Autodesk Inventor part; units mm, degrees
(part 4 of 13)
  arc A1197 (1.0789, 60.921) -> (1.0789, 60.795) centre (1.0789, 60.858) ccw
  line L1196 (7.637, 60.795) -> (7.7628, 60.795)
  arc A1198 (7.7628, 60.795) -> (7.7628, 60.921) centre (7.7628, 60.858) ccw
  line L1197 (7.7628, 60.921) -> (7.637, 60.921)
  arc A1199 (7.637, 60.921) -> (7.637, 60.795) centre (7.637, 60.858) ccw
  line L1198 (8.7151, 60.795) -> (17.121, 60.795)
  arc A1200 (17.121, 60.795) -> (17.121, 60.921) centre (17.121, 60.858) ccw
  line L1199 (17.121, 60.921) -> (8.7151, 60.921)
  arc A1201 (8.7151, 60.921) -> (8.7151, 60.795) centre (8.7151, 60.858) ccw
  line L1200 (1.0789, 60.921) -> (6.8108, 60.921)
  arc A1202 (6.8108, 60.921) -> (6.8108, 61.047) centre (6.8108, 60.984) ccw
  line L1201 (6.8108, 61.047) -> (1.0789, 61.047)
  arc A1203 (1.0789, 61.047) -> (1.0789, 60.921) centre (1.0789, 60.984) ccw
  line L1202 (7.637, 60.921) -> (7.7628, 60.921)
  arc A1204 (7.7628, 60.921) -> (7.7628, 61.047) centre (7.7628, 60.984) ccw
  line L1203 (7.7628, 61.047) -> (7.637, 61.047)
  arc A1205 (7.637, 61.047) -> (7.637, 60.921) centre (7.637, 60.984) ccw
  line L1204 (8.5891, 60.921) -> (17.121, 60.921)
  arc A1206 (17.121, 60.921) -> (17.121, 61.047) centre (17.121, 60.984) ccw
  line L1205 (17.121, 61.047) -> (8.5891, 61.047)
  arc A1207 (8.5891, 61.047) -> (8.5891, 60.921) centre (8.5891, 60.984) ccw
  line L1206 (1.0789, 61.047) -> (6.9527, 61.047)
  arc A1208 (6.9527, 61.047) -> (6.9527, 61.173) centre (6.9527, 61.11) ccw
  line L1207 (6.9527, 61.173) -> (1.0789, 61.173)
  arc A1209 (1.0789, 61.173) -> (1.0789, 61.047) centre (1.0789, 61.11) ccw
  line L1208 (7.637, 61.047) -> (7.7628, 61.047)
  arc A1210 (7.7628, 61.047) -> (7.7628, 61.173) centre (7.7628, 61.11) ccw
  line L1209 (7.7628, 61.173) -> (7.637, 61.173)
  arc A1211 (7.637, 61.173) -> (7.637, 61.047) centre (7.637, 61.11) ccw
  line L1210 (8.4473, 61.047) -> (17.121, 61.047)
  arc A1212 (17.121, 61.047) -> (17.121, 61.173) centre (17.121, 61.11) ccw
  line L1211 (17.121, 61.173) -> (8.4473, 61.173)
  arc A1213 (8.4473, 61.173) -> (8.4473, 61.047) centre (8.4473, 61.11) ccw
  line L1212 (1.0789, 61.173) -> (7.2569, 61.173)
  arc A1214 (7.2569, 61.173) -> (7.2569, 61.299) centre (7.2569, 61.236) ccw
  line L1213 (7.2569, 61.299) -> (1.0789, 61.299)
  arc A1215 (1.0789, 61.299) -> (1.0789, 61.173) centre (1.0789, 61.236) ccw
  line L1214 (7.637, 61.173) -> (7.7628, 61.173)
  arc A1216 (7.7628, 61.173) -> (7.7628, 61.299) centre (7.7628, 61.236) ccw
  line L1215 (7.7628, 61.299) -> (7.637, 61.299)
  arc A1217 (7.637, 61.299) -> (7.637, 61.173) centre (7.637, 61.236) ccw
  line L1216 (8.1431, 61.173) -> (17.121, 61.173)
  arc A1218 (17.121, 61.173) -> (17.121, 61.299) centre (17.121, 61.236) ccw
  line L1217 (17.121, 61.299) -> (8.1431, 61.299)
  arc A1219 (8.1431, 61.299) -> (8.1431, 61.173) centre (8.1431, 61.236) ccw
  line L1218 (1.0789, 61.299) -> (17.121, 61.299)
  arc A1220 (17.121, 61.299) -> (17.121, 61.425) centre (17.121, 61.362) ccw
  line L1219 (17.121, 61.425) -> (1.0789, 61.425)
  arc A1221 (1.0789, 61.425) -> (1.0789, 61.299) centre (1.0789, 61.362) ccw
  line L1220 (1.0789, 61.425) -> (17.121, 61.425)
  arc A1222 (17.121, 61.425) -> (17.121, 61.551) centre (17.121, 61.488) ccw
  line L1221 (17.121, 61.551) -> (1.0789, 61.551)
  arc A1223 (1.0789, 61.551) -> (1.0789, 61.425) centre (1.0789, 61.488) ccw
  line L1222 (1.0789, 61.551) -> (17.121, 61.551)
  arc A1224 (17.121, 61.551) -> (17.121, 61.677) centre (17.121, 61.614) ccw
  line L1223 (17.121, 61.677) -> (1.0789, 61.677)
  arc A1225 (1.0789, 61.677) -> (1.0789, 61.551) centre (1.0789, 61.614) ccw
  line L1224 (1.0789, 61.677) -> (17.121, 61.677)
  arc A1226 (17.121, 61.677) -> (17.121, 61.803) centre (17.121, 61.74) ccw
  line L1225 (17.121, 61.803) -> (1.0789, 61.803)
  arc A1227 (1.0789, 61.803) -> (1.0789, 61.677) centre (1.0789, 61.74) ccw
  line L1226 (1.0789, 61.803) -> (17.121, 61.803)
  arc A1228 (17.121, 61.803) -> (17.121, 61.929) centre (17.121, 61.866) ccw
  line L1227 (17.121, 61.929) -> (1.0789, 61.929)
  arc A1229 (1.0789, 61.929) -> (1.0789, 61.803) centre (1.0789, 61.866) ccw
  line L1228 (1.0789, 61.929) -> (17.121, 61.929)
  arc A1230 (17.121, 61.929) -> (17.121, 62.055) centre (17.121, 61.992) ccw
  line L1229 (17.121, 62.055) -> (1.0789, 62.055)
  arc A1231 (1.0789, 62.055) -> (1.0789, 61.929) centre (1.0789, 61.992) ccw
  line L1230 (1.0789, 62.055) -> (17.121, 62.055)
  arc A1232 (17.121, 62.055) -> (17.121, 62.181) centre (17.121, 62.118) ccw
  line L1231 (17.121, 62.181) -> (1.0789, 62.181)
  arc A1233 (1.0789, 62.181) -> (1.0789, 62.055) centre (1.0789, 62.118) ccw
  line L1232 (1.0789, 62.181) -> (17.121, 62.181)
  arc A1234 (17.121, 62.181) -> (17.121, 62.307) centre (17.121, 62.244) ccw
  line L1233 (17.121, 62.307) -> (1.0789, 62.307)
  arc A1235 (1.0789, 62.307) -> (1.0789, 62.181) centre (1.0789, 62.244) ccw
  line L1234 (1.0789, 62.307) -> (17.121, 62.307)
  arc A1236 (17.121, 62.307) -> (17.121, 62.433) centre (17.121, 62.37) ccw
  line L1235 (17.121, 62.433) -> (1.0789, 62.433)
  arc A1237 (1.0789, 62.433) -> (1.0789, 62.307) centre (1.0789, 62.37) ccw
  line L1236 (1.0789, 62.433) -> (17.121, 62.433)
  arc A1238 (17.121, 62.433) -> (17.121, 62.559) centre (17.121, 62.496) ccw
  line L1237 (17.121, 62.559) -> (1.0789, 62.559)
  arc A1239 (1.0789, 62.559) -> (1.0789, 62.433) centre (1.0789, 62.496) ccw
  line L1238 (1.0789, 62.559) -> (17.121, 62.559)
  arc A1240 (17.121, 62.559) -> (17.121, 62.685) centre (17.121, 62.622) ccw
  line L1239 (17.121, 62.685) -> (1.0789, 62.685)
  arc A1241 (1.0789, 62.685) -> (1.0789, 62.559) centre (1.0789, 62.622) ccw
  line L1240 (1.0789, 62.685) -> (17.121, 62.685)
  arc A1242 (17.121, 62.685) -> (17.121, 62.811) centre (17.121, 62.748) ccw
  line L1241 (17.121, 62.811) -> (1.0789, 62.811)
  arc A1243 (1.0789, 62.811) -> (1.0789, 62.685) centre (1.0789, 62.748) ccw
  line L1242 (1.0789, 62.811) -> (17.121, 62.811)
  arc A1244 (17.121, 62.811) -> (17.121, 62.937) centre (17.121, 62.874) ccw
  line L1243 (17.121, 62.937) -> (1.0789, 62.937)
  arc A1245 (1.0789, 62.937) -> (1.0789, 62.811) centre (1.0789, 62.874) ccw
  line L1244 (1.0789, 62.937) -> (17.121, 62.937)
  arc A1246 (17.121, 62.937) -> (17.121, 63.063) centre (17.121, 63) ccw
  line L1245 (17.121, 63.063) -> (1.0789, 63.063)
  arc A1247 (1.0789, 63.063) -> (1.0789, 62.937) centre (1.0789, 63) ccw
  line L1246 (1.0789, 63.063) -> (17.121, 63.063)
  arc A1248 (17.121, 63.063) -> (17.121, 63.189) centre (17.121, 63.126) ccw
  line L1247 (17.121, 63.189) -> (1.0789, 63.189)
  arc A1249 (1.0789, 63.189) -> (1.0789, 63.063) centre (1.0789, 63.126) ccw
  line L1248 (17.058, 63.221) -> (17.058, 1.0789)
  arc A1250 (17.058, 1.0789) -> (17.184, 1.0789) centre (17.121, 1.0789) ccw
  line L1249 (17.184, 1.0789) -> (17.184, 63.221)
  arc A1251 (17.184, 63.221) -> (17.058, 63.221) centre (17.121, 63.221) ccw
  line L1250 (17.121, 1.1419) -> (1.0789, 1.1419)
  arc A1252 (1.0789, 1.1419) -> (1.0789, 1.0159) centre (1.0789, 1.0789) ccw
  line L1251 (1.0789, 1.0159) -> (17.121, 1.0159)
  arc A1253 (17.121, 1.0159) -> (17.121, 1.1419) centre (17.121, 1.0789) ccw
  line L1252 (1.1419, 1.0789) -> (1.1419, 63.221)
  arc A1254 (1.1419, 63.221) -> (1.0159, 63.221) centre (1.0789, 63.221) ccw
  line L1253 (1.0159, 63.221) -> (1.0159, 1.0789)
  arc A1255 (1.0159, 1.0789) -> (1.1419, 1.0789) centre (1.0789, 1.0789) ccw
  line L1254 (1.0789, 63.158) -> (17.121, 63.158)
  arc A1256 (17.121, 63.158) -> (17.121, 63.284) centre (17.121, 63.221) ccw
  line L1255 (17.121, 63.284) -> (1.0789, 63.284)
  arc A1257 (1.0789, 63.284) -> (1.0789, 63.158) centre (1.0789, 63.221) ccw
  line L1256 (7.428, 58.51) -> (7.637, 58.51)
  arc A1258 (7.637, 58.51) -> (7.637, 58.636) centre (7.637, 58.573) ccw
  line L1257 (7.637, 58.636) -> (7.428, 58.636)
  arc A1259 (7.428, 58.636) -> (7.428, 58.51) centre (7.428, 58.573) ccw
  line L1258 (7.7, 58.573) -> (7.7, 59.8765)
  arc A1260 (7.7, 59.8765) -> (7.574, 59.8765) centre (7.637, 59.8765) ccw
  line L1259 (7.574, 59.8765) -> (7.574, 58.573)
  arc A1261 (7.574, 58.573) -> (7.7, 58.573) centre (7.637, 58.573) ccw
  line L1260 (7.637, 59.8135) -> (7.7628, 59.8135)
  arc A1262 (7.7628, 59.8135) -> (7.7628, 59.9395) centre (7.7628, 59.8765) ccw
  line L1261 (7.7628, 59.9395) -> (7.637, 59.9395)
  arc A1263 (7.637, 59.9395) -> (7.637, 59.8135) centre (7.637, 59.8765) ccw
  line L1262 (7.6998, 59.8765) -> (7.6998, 58.573)
  arc A1264 (7.6998, 58.573) -> (7.8258, 58.573) centre (7.7628, 58.573) ccw
  line L1263 (7.8258, 58.573) -> (7.8258, 59.8765)
  arc A1265 (7.8258, 59.8765) -> (7.6998, 59.8765) centre (7.7628, 59.8765) ccw
  line L1264 (7.7628, 58.51) -> (7.9719, 58.51)
  arc A1266 (7.9719, 58.51) -> (7.9719, 58.636) centre (7.9719, 58.573) ccw
  line L1265 (7.9719, 58.636) -> (7.7628, 58.636)
  arc A1267 (7.7628, 58.636) -> (7.7628, 58.51) centre (7.7628, 58.573) ccw
  line L1266 (7.996, 58.5148) -> (8.4984, 58.7229)
  arc A1268 (8.4984, 58.7229) -> (8.4502, 58.8393) centre (8.4743, 58.7811) ccw
  line L1267 (8.4502, 58.8393) -> (7.9478, 58.6312)
  arc A1269 (7.9478, 58.6312) -> (7.996, 58.5148) centre (7.9719, 58.573) ccw
  line L1268 (8.5188, 58.7366) -> (8.9033, 59.1211)
  arc A1270 (8.9033, 59.1211) -> (8.8143, 59.2101) centre (8.8588, 59.1656) ccw
  line L1269 (8.8143, 59.2101) -> (8.4298, 58.8256)
  arc A1271 (8.4298, 58.8256) -> (8.5188, 58.7366) centre (8.4743, 58.7811) ccw
  line L1270 (8.917, 59.1415) -> (9.1251, 59.6439)
  arc A1272 (9.1251, 59.6439) -> (9.0087, 59.6921) centre (9.0669, 59.668) ccw
  line L1271 (9.0087, 59.6921) -> (8.8006, 59.1897)
  arc A1273 (8.8006, 59.1897) -> (8.917, 59.1415) centre (8.8588, 59.1656) ccw
  line L1272 (9.1299, 59.668) -> (9.1299, 59.877)
  arc A1274 (9.1299, 59.877) -> (9.0039, 59.877) centre (9.0669, 59.877) ccw
  line L1273 (9.0039, 59.877) -> (9.0039, 59.668)
  arc A1275 (9.0039, 59.668) -> (9.1299, 59.668) centre (9.0669, 59.668) ccw
  line L1274 (9.0669, 59.94) -> (7.7634, 59.94)
  arc A1276 (7.7634, 59.94) -> (7.7634, 59.814) centre (7.7634, 59.877) ccw
  line L1275 (7.7634, 59.814) -> (9.0669, 59.814)
  arc A1277 (9.0669, 59.814) -> (9.0669, 59.94) centre (9.0669, 59.877) ccw
  line L1276 (7.8264, 59.877) -> (7.8264, 60.0028)
  arc A1278 (7.8264, 60.0028) -> (7.7004, 60.0028) centre (7.7634, 60.0028) ccw
  line L1277 (7.7004, 60.0028) -> (7.7004, 59.877)
  arc A1279 (7.7004, 59.877) -> (7.8264, 59.877) centre (7.7634, 59.877) ccw
  line L1278 (7.7634, 59.9398) -> (9.0669, 59.9398)
  arc A1280 (9.0669, 59.9398) -> (9.0669, 60.0658) centre (9.0669, 60.0028) ccw
  line L1279 (9.0669, 60.0658) -> (7.7634, 60.0658)
  arc A1281 (7.7634, 60.0658) -> (7.7634, 59.9398) centre (7.7634, 60.0028) ccw
  line L1280 (9.1299, 60.0028) -> (9.1299, 60.2119)
  arc A1282 (9.1299, 60.2119) -> (9.0039, 60.2119) centre (9.0669, 60.2119) ccw
  line L1281 (9.0039, 60.2119) -> (9.0039, 60.0028)
  arc A1283 (9.0039, 60.0028) -> (9.1299, 60.0028) centre (9.0669, 60.0028) ccw
  line L1282 (9.1251, 60.236) -> (8.917, 60.7384)
  arc A1284 (8.917, 60.7384) -> (8.8006, 60.6902) centre (8.8588, 60.7143) ccw
  line L1283 (8.8006, 60.6902) -> (9.0087, 60.1878)
  arc A1285 (9.0087, 60.1878) -> (9.1251, 60.236) centre (9.0669, 60.2119) ccw
  line L1284 (8.9033, 60.7588) -> (8.5188, 61.1433)
  arc A1286 (8.5188, 61.1433) -> (8.4298, 61.0543) centre (8.4743, 61.0988) ccw
  line L1285 (8.4298, 61.0543) -> (8.8143, 60.6698)
  arc A1287 (8.8143, 60.6698) -> (8.9033, 60.7588) centre (8.8588, 60.7143) ccw
  line L1286 (8.4984, 61.157) -> (7.996, 61.3651)
  arc A1288 (7.996, 61.3651) -> (7.9478, 61.2487) centre (7.9719, 61.3069) ccw
  line L1287 (7.9478, 61.2487) -> (8.4502, 61.0406)
  arc A1289 (8.4502, 61.0406) -> (8.4984, 61.157) centre (8.4743, 61.0988) ccw
  line L1288 (7.9719, 61.3699) -> (7.7628, 61.3699)
  arc A1290 (7.7628, 61.3699) -> (7.7628, 61.2439) centre (7.7628, 61.3069) ccw
  line L1289 (7.7628, 61.2439) -> (7.9719, 61.2439)
  arc A1291 (7.9719, 61.2439) -> (7.9719, 61.3699) centre (7.9719, 61.3069) ccw
  line L1290 (7.6998, 61.3069) -> (7.6998, 60.0034)
  arc A1292 (7.6998, 60.0034) -> (7.8258, 60.0034) centre (7.7628, 60.0034) ccw
  line L1291 (7.8258, 60.0034) -> (7.8258, 61.3069)
  arc A1293 (7.8258, 61.3069) -> (7.6998, 61.3069) centre (7.7628, 61.3069) ccw
  line L1292 (7.7628, 60.0664) -> (7.637, 60.0664)
  arc A1294 (7.637, 60.0664) -> (7.637, 59.9404) centre (7.637, 60.0034) ccw
  line L1293 (7.637, 59.9404) -> (7.7628, 59.9404)
  arc A1295 (7.7628, 59.9404) -> (7.7628, 60.0664) centre (7.7628, 60.0034) ccw
  line L1294 (7.7, 60.0034) -> (7.7, 61.3069)
  arc A1296 (7.7, 61.3069) -> (7.574, 61.3069) centre (7.637, 61.3069) ccw
  line L1295 (7.574, 61.3069) -> (7.574, 60.0034)
  arc A1297 (7.574, 60.0034) -> (7.7, 60.0034) centre (7.637, 60.0034) ccw
  line L1296 (7.637, 61.3699) -> (7.428, 61.3699)
  arc A1298 (7.428, 61.3699) -> (7.428, 61.2439) centre (7.428, 61.3069) ccw
  line L1297 (7.428, 61.2439) -> (7.637, 61.2439)
  arc A1299 (7.637, 61.2439) -> (7.637, 61.3699) centre (7.637, 61.3069) ccw
  line L1298 (7.4039, 61.3651) -> (6.9015, 61.157)
  arc A1300 (6.9015, 61.157) -> (6.9497, 61.0406) centre (6.9256, 61.0988) ccw
  line L1299 (6.9497, 61.0406) -> (7.4521, 61.2487)
  arc A1301 (7.4521, 61.2487) -> (7.4039, 61.3651) centre (7.428, 61.3069) ccw
  line L1300 (6.8811, 61.1433) -> (6.4966, 60.7588)
  arc A1302 (6.4966, 60.7588) -> (6.5856, 60.6698) centre (6.5411, 60.7143) ccw
  line L1301 (6.5856, 60.6698) -> (6.9701, 61.0543)
  arc A1303 (6.9701, 61.0543) -> (6.8811, 61.1433) centre (6.9256, 61.0988) ccw
  line L1302 (6.4829, 60.7384) -> (6.2748, 60.236)
  arc A1304 (6.2748, 60.236) -> (6.3912, 60.1878) centre (6.333, 60.2119) ccw
  line L1303 (6.3912, 60.1878) -> (6.5993, 60.6902)
  arc A1305 (6.5993, 60.6902) -> (6.4829, 60.7384) centre (6.5411, 60.7143) ccw
  line L1304 (6.27, 60.2119) -> (6.27, 60.0028)
  arc A1306 (6.27, 60.0028) -> (6.396, 60.0028) centre (6.333, 60.0028) ccw
  line L1305 (6.396, 60.0028) -> (6.396, 60.2119)
  arc A1307 (6.396, 60.2119) -> (6.27, 60.2119) centre (6.333, 60.2119) ccw
  line L1306 (6.333, 59.9398) -> (7.6365, 59.9398)
  arc A1308 (7.6365, 59.9398) -> (7.6365, 60.0658) centre (7.6365, 60.0028) ccw
  line L1307 (7.6365, 60.0658) -> (6.333, 60.0658)
  arc A1309 (6.333, 60.0658) -> (6.333, 59.9398) centre (6.333, 60.0028) ccw
  line L1308 (7.5735, 60.0028) -> (7.5735, 59.877)
  arc A1310 (7.5735, 59.877) -> (7.6995, 59.877) centre (7.6365, 59.877) ccw
  line L1309 (7.6995, 59.877) -> (7.6995, 60.0028)
  arc A1311 (7.6995, 60.0028) -> (7.5735, 60.0028) centre (7.6365, 60.0028) ccw
  line L1310 (7.6365, 59.94) -> (6.333, 59.94)
  arc A1312 (6.333, 59.94) -> (6.333, 59.814) centre (6.333, 59.877) ccw
  line L1311 (6.333, 59.814) -> (7.6365, 59.814)
  arc A1313 (7.6365, 59.814) -> (7.6365, 59.94) centre (7.6365, 59.877) ccw
  line L1312 (6.27, 59.877) -> (6.27, 59.668)
  arc A1314 (6.27, 59.668) -> (6.396, 59.668) centre (6.333, 59.668) ccw
  line L1313 (6.396, 59.668) -> (6.396, 59.877)
  arc A1315 (6.396, 59.877) -> (6.27, 59.877) centre (6.333, 59.877) ccw
  line L1314 (6.2748, 59.6439) -> (6.4829, 59.1415)
  arc A1316 (6.4829, 59.1415) -> (6.5993, 59.1897) centre (6.5411, 59.1656) ccw
  line L1315 (6.5993, 59.1897) -> (6.3912, 59.6921)
  arc A1317 (6.3912, 59.6921) -> (6.2748, 59.6439) centre (6.333, 59.668) ccw
  line L1316 (6.4966, 59.1211) -> (6.8811, 58.7366)
  arc A1318 (6.8811, 58.7366) -> (6.9701, 58.8256) centre (6.9256, 58.7811) ccw
  line L1317 (6.9701, 58.8256) -> (6.5856, 59.2101)
  arc A1319 (6.5856, 59.2101) -> (6.4966, 59.1211) centre (6.5411, 59.1656) ccw
  line L1318 (6.9015, 58.7229) -> (7.4039, 58.5148)
  arc A1320 (7.4039, 58.5148) -> (7.4521, 58.6312) centre (7.428, 58.573) ccw
  line L1319 (7.4521, 58.6312) -> (6.9497, 58.8393)
  arc A1321 (6.9497, 58.8393) -> (6.9015, 58.7229) centre (6.9256, 58.7811) ccw
  line L1320 (9.0283, 54.6082) -> (9.0283, 55.1117)
  arc A1322 (9.0283, 55.1117) -> (8.9023, 55.1117) centre (8.9653, 55.1117) ccw
  line L1321 (8.9023, 55.1117) -> (8.9023, 54.6082)
  arc A1323 (8.9023, 54.6082) -> (9.0283, 54.6082) centre (8.9653, 54.6082) ccw
  line L1322 (9.0235, 55.1358) -> (8.8309, 55.6008)
  arc A1324 (8.8309, 55.6008) -> (8.7145, 55.5526) centre (8.7727, 55.5767) ccw
  line L1323 (8.7145, 55.5526) -> (8.9071, 55.0876)
  arc A1325 (8.9071, 55.0876) -> (9.0235, 55.1358) centre (8.9653, 55.1117) ccw
  line L1324 (8.8172, 55.6212) -> (8.4612, 55.9772)
  arc A1326 (8.4612, 55.9772) -> (8.3722, 55.8882) centre (8.4167, 55.9327) ccw
  line L1325 (8.3722, 55.8882) -> (8.7282, 55.5322)
  arc A1327 (8.7282, 55.5322) -> (8.8172, 55.6212) centre (8.7727, 55.5767) ccw
  line L1326 (8.4408, 55.9909) -> (7.9758, 56.1835)
  arc A1328 (7.9758, 56.1835) -> (7.9276, 56.0671) centre (7.9517, 56.1253) ccw
  line L1327 (7.9276, 56.0671) -> (8.3926, 55.8745)
  arc A1329 (8.3926, 55.8745) -> (8.4408, 55.9909) centre (8.4167, 55.9327) ccw
  line L1328 (7.9517, 56.1883) -> (7.4482, 56.1883)
  arc A1330 (7.4482, 56.1883) -> (7.4482, 56.0623) centre (7.4482, 56.1253) ccw
  line L1329 (7.4482, 56.0623) -> (7.9517, 56.0623)
  arc A1331 (7.9517, 56.0623) -> (7.9517, 56.1883) centre (7.9517, 56.1253) ccw
  line L1330 (7.4241, 56.1835) -> (6.9591, 55.9909)
  arc A1332 (6.9591, 55.9909) -> (7.0073, 55.8745) centre (6.9832, 55.9327) ccw
  line L1331 (7.0073, 55.8745) -> (7.4723, 56.0671)
  arc A1333 (7.4723, 56.0671) -> (7.4241, 56.1835) centre (7.4482, 56.1253) ccw
  line L1332 (6.9387, 55.9772) -> (6.5827, 55.6212)
  arc A1334 (6.5827, 55.6212) -> (6.6717, 55.5322) centre (6.6272, 55.5767) ccw
  line L1333 (6.6717, 55.5322) -> (7.0277, 55.8882)
  arc A1335 (7.0277, 55.8882) -> (6.9387, 55.9772) centre (6.9832, 55.9327) ccw
  line L1334 (6.569, 55.6008) -> (6.3764, 55.1358)
  arc A1336 (6.3764, 55.1358) -> (6.4928, 55.0876) centre (6.4346, 55.1117) ccw
  line L1335 (6.4928, 55.0876) -> (6.6854, 55.5526)
  arc A1337 (6.6854, 55.5526) -> (6.569, 55.6008) centre (6.6272, 55.5767) ccw
  line L1336 (6.3716, 55.1117) -> (6.3716, 54.6082)
  arc A1338 (6.3716, 54.6082) -> (6.4976, 54.6082) centre (6.4346, 54.6082) ccw
  line L1337 (6.4976, 54.6082) -> (6.4976, 55.1117)
  arc A1339 (6.4976, 55.1117) -> (6.3716, 55.1117) centre (6.4346, 55.1117) ccw
  line L1338 (6.3764, 54.5841) -> (6.569, 54.1191)
  arc A1340 (6.569, 54.1191) -> (6.6854, 54.1673) centre (6.6272, 54.1432) ccw
  line L1339 (6.6854, 54.1673) -> (6.4928, 54.6323)
  arc A1341 (6.4928, 54.6323) -> (6.3764, 54.5841) centre (6.4346, 54.6082) ccw
  line L1340 (6.5827, 54.0987) -> (6.9387, 53.7427)
  arc A1342 (6.9387, 53.7427) -> (7.0277, 53.8317) centre (6.9832, 53.7872) ccw
  line L1341 (7.0277, 53.8317) -> (6.6717, 54.1877)
  arc A1343 (6.6717, 54.1877) -> (6.5827, 54.0987) centre (6.6272, 54.1432) ccw
  line L1342 (6.9591, 53.729) -> (7.4241, 53.5364)
  arc A1344 (7.4241, 53.5364) -> (7.4723, 53.6528) centre (7.4482, 53.5946) ccw
  line L1343 (7.4723, 53.6528) -> (7.0073, 53.8454)
  arc A1345 (7.0073, 53.8454) -> (6.9591, 53.729) centre (6.9832, 53.7872) ccw
  line L1344 (7.4482, 53.5316) -> (7.9517, 53.5316)
  arc A1346 (7.9517, 53.5316) -> (7.9517, 53.6576) centre (7.9517, 53.5946) ccw
  line L1345 (7.9517, 53.6576) -> (7.4482, 53.6576)
  arc A1347 (7.4482, 53.6576) -> (7.4482, 53.5316) centre (7.4482, 53.5946) ccw
  line L1346 (7.9758, 53.5364) -> (8.4408, 53.729)
  arc A1348 (8.4408, 53.729) -> (8.3926, 53.8454) centre (8.4167, 53.7872) ccw
  line L1347 (8.3926, 53.8454) -> (7.9276, 53.6528)
  arc A1349 (7.9276, 53.6528) -> (7.9758, 53.5364) centre (7.9517, 53.5946) ccw
  line L1348 (8.4612, 53.7427) -> (8.8172, 54.0987)
  arc A1350 (8.8172, 54.0987) -> (8.7282, 54.1877) centre (8.7727, 54.1432) ccw
  line L1349 (8.7282, 54.1877) -> (8.3722, 53.8317)
  arc A1351 (8.3722, 53.8317) -> (8.4612, 53.7427) centre (8.4167, 53.7872) ccw
  line L1350 (8.8309, 54.1191) -> (9.0235, 54.5841)
  arc A1352 (9.0235, 54.5841) -> (8.9071, 54.6323) centre (8.9653, 54.6082) ccw
  line L1351 (8.9071, 54.6323) -> (8.7145, 54.1673)
  arc A1353 (8.7145, 54.1673) -> (8.8309, 54.1191) centre (8.7727, 54.1432) ccw
  line L1352 (7.428, 38.19) -> (7.637, 38.19)
  arc A1354 (7.637, 38.19) -> (7.637, 38.316) centre (7.637, 38.253) ccw
  line L1353 (7.637, 38.316) -> (7.428, 38.316)
  arc A1355 (7.428, 38.316) -> (7.428, 38.19) centre (7.428, 38.253) ccw
  line L1354 (7.7, 38.253) -> (7.7, 39.5565)
  arc A1356 (7.7, 39.5565) -> (7.574, 39.5565) centre (7.637, 39.5565) ccw
  line L1355 (7.574, 39.5565) -> (7.574, 38.253)
  arc A1357 (7.574, 38.253) -> (7.7, 38.253) centre (7.637, 38.253) ccw
  line L1356 (7.637, 39.4935) -> (7.7628, 39.4935)
  arc A1358 (7.7628, 39.4935) -> (7.7628, 39.6195) centre (7.7628, 39.5565) ccw
  line L1357 (7.7628, 39.6195) -> (7.637, 39.6195)
  arc A1359 (7.637, 39.6195) -> (7.637, 39.4935) centre (7.637, 39.5565) ccw
  line L1358 (7.6998, 39.5565) -> (7.6998, 38.253)
  arc A1360 (7.6998, 38.253) -> (7.8258, 38.253) centre (7.7628, 38.253) ccw
  line L1359 (7.8258, 38.253) -> (7.8258, 39.5565)
  arc A1361 (7.8258, 39.5565) -> (7.6998, 39.5565) centre (7.7628, 39.5565) ccw
  line L1360 (7.7628, 38.19) -> (7.9719, 38.19)
  arc A1362 (7.9719, 38.19) -> (7.9719, 38.316) centre (7.9719, 38.253) ccw
  line L1361 (7.9719, 38.316) -> (7.7628, 38.316)
  arc A1363 (7.7628, 38.316) -> (7.7628, 38.19) centre (7.7628, 38.253) ccw
  line L1362 (7.996, 38.1948) -> (8.4984, 38.4029)
  arc A1364 (8.4984, 38.4029) -> (8.4502, 38.5193) centre (8.4743, 38.4611) ccw
  line L1363 (8.4502, 38.5193) -> (7.9478, 38.3112)
  arc A1365 (7.9478, 38.3112) -> (7.996, 38.1948) centre (7.9719, 38.253) ccw
  line L1364 (8.5188, 38.4166) -> (8.9033, 38.8011)
  arc A1366 (8.9033, 38.8011) -> (8.8143, 38.8901) centre (8.8588, 38.8456) ccw
  line L1365 (8.8143, 38.8901) -> (8.4298, 38.5056)
  arc A1367 (8.4298, 38.5056) -> (8.5188, 38.4166) centre (8.4743, 38.4611) ccw
  line L1366 (8.917, 38.8215) -> (9.1251, 39.3239)
  arc A1368 (9.1251, 39.3239) -> (9.0087, 39.3721) centre (9.0669, 39.348) ccw
  line L1367 (9.0087, 39.3721) -> (8.8006, 38.8697)
  arc A1369 (8.8006, 38.8697) -> (8.917, 38.8215) centre (8.8588, 38.8456) ccw
  line L1368 (9.1299, 39.348) -> (9.1299, 39.557)
  arc A1370 (9.1299, 39.557) -> (9.0039, 39.557) centre (9.0669, 39.557) ccw
  line L1369 (9.0039, 39.557) -> (9.0039, 39.348)
  arc A1371 (9.0039, 39.348) -> (9.1299, 39.348) centre (9.0669, 39.348) ccw
  line L1370 (9.0669, 39.62) -> (7.7634, 39.62)
  arc A1372 (7.7634, 39.62) -> (7.7634, 39.494) centre (7.7634, 39.557) ccw
  line L1371 (7.7634, 39.494) -> (9.0669, 39.494)
  arc A1373 (9.0669, 39.494) -> (9.0669, 39.62) centre (9.0669, 39.557) ccw
  line L1372 (7.8264, 39.557) -> (7.8264, 39.6828)
  arc A1374 (7.8264, 39.6828) -> (7.7004, 39.6828) centre (7.7634, 39.6828) ccw
  line L1373 (7.7004, 39.6828) -> (7.7004, 39.557)
  arc A1375 (7.7004, 39.557) -> (7.8264, 39.557) centre (7.7634, 39.557) ccw
  line L1374 (7.7634, 39.6198) -> (9.0669, 39.6198)
  arc A1376 (9.0669, 39.6198) -> (9.0669, 39.7458) centre (9.0669, 39.6828) ccw
  line L1375 (9.0669, 39.7458) -> (7.7634, 39.7458)
  arc A1377 (7.7634, 39.7458) -> (7.7634, 39.6198) centre (7.7634, 39.6828) ccw
  line L1376 (9.1299, 39.6828) -> (9.1299, 39.8919)
  arc A1378 (9.1299, 39.8919) -> (9.0039, 39.8919) centre (9.0669, 39.8919) ccw
  line L1377 (9.0039, 39.8919) -> (9.0039, 39.6828)
  arc A1379 (9.0039, 39.6828) -> (9.1299, 39.6828) centre (9.0669, 39.6828) ccw
  line L1378 (9.1251, 39.916) -> (8.917, 40.4184)
  arc A1380 (8.917, 40.4184) -> (8.8006, 40.3702) centre (8.8588, 40.3943) ccw
  line L1379 (8.8006, 40.3702) -> (9.0087, 39.8678)
  arc A1381 (9.0087, 39.8678) -> (9.1251, 39.916) centre (9.0669, 39.8919) ccw
  line L1380 (8.9033, 40.4388) -> (8.5188, 40.8233)
  arc A1382 (8.5188, 40.8233) -> (8.4298, 40.7343) centre (8.4743, 40.7788) ccw
  line L1381 (8.4298, 40.7343) -> (8.8143, 40.3498)
  arc A1383 (8.8143, 40.3498) -> (8.9033, 40.4388) centre (8.8588, 40.3943) ccw
  line L1382 (8.4984, 40.837) -> (7.996, 41.0451)
  arc A1384 (7.996, 41.0451) -> (7.9478, 40.9287) centre (7.9719, 40.9869) ccw
  line L1383 (7.9478, 40.9287) -> (8.4502, 40.7206)
  arc A1385 (8.4502, 40.7206) -> (8.4984, 40.837) centre (8.4743, 40.7788) ccw
  line L1384 (7.9719, 41.0499) -> (7.7628, 41.0499)
  arc A1386 (7.7628, 41.0499) -> (7.7628, 40.9239) centre (7.7628, 40.9869) ccw
  line L1385 (7.7628, 40.9239) -> (7.9719, 40.9239)
  arc A1387 (7.9719, 40.9239) -> (7.9719, 41.0499) centre (7.9719, 40.9869) ccw
  line L1386 (7.6998, 40.9869) -> (7.6998, 39.6834)
  arc A1388 (7.6998, 39.6834) -> (7.8258, 39.6834) centre (7.7628, 39.6834) ccw
  line L1387 (7.8258, 39.6834) -> (7.8258, 40.9869)
  arc A1389 (7.8258, 40.9869) -> (7.6998, 40.9869) centre (7.7628, 40.9869) ccw
  line L1388 (7.7628, 39.7464) -> (7.637, 39.7464)
  arc A1390 (7.637, 39.7464) -> (7.637, 39.6204) centre (7.637, 39.6834) ccw
  line L1389 (7.637, 39.6204) -> (7.7628, 39.6204)
  arc A1391 (7.7628, 39.6204) -> (7.7628, 39.7464) centre (7.7628, 39.6834) ccw
  line L1390 (7.7, 39.6834) -> (7.7, 40.9869)
  arc A1392 (7.7, 40.9869) -> (7.574, 40.9869) centre (7.637, 40.9869) ccw
  line L1391 (7.574, 40.9869) -> (7.574, 39.6834)
  arc A1393 (7.574, 39.6834) -> (7.7, 39.6834) centre (7.637, 39.6834) ccw
  line L1392 (7.637, 41.0499) -> (7.428, 41.0499)
  arc A1394 (7.428, 41.0499) -> (7.428, 40.9239) centre (7.428, 40.9869) ccw
  line L1393 (7.428, 40.9239) -> (7.637, 40.9239)
  arc A1395 (7.637, 40.9239) -> (7.637, 41.0499) centre (7.637, 40.9869) ccw
  line L1394 (7.4039, 41.0451) -> (6.9015, 40.837)
  arc A1396 (6.9015, 40.837) -> (6.9497, 40.7206) centre (6.9256, 40.7788) ccw
  line L1395 (6.9497, 40.7206) -> (7.4521, 40.9287)
  arc A1397 (7.4521, 40.9287) -> (7.4039, 41.0451) centre (7.428, 40.9869) ccw
  line L1396 (6.8811, 40.8233) -> (6.4966, 40.4388)
  arc A1398 (6.4966, 40.4388) -> (6.5856, 40.3498) centre (6.5411, 40.3943) ccw
  line L1397 (6.5856, 40.3498) -> (6.9701, 40.7343)
  arc A1399 (6.9701, 40.7343) -> (6.8811, 40.8233) centre (6.9256, 40.7788) ccw
  line L1398 (6.4829, 40.4184) -> (6.2748, 39.916)
  arc A1400 (6.2748, 39.916) -> (6.3912, 39.8678) centre (6.333, 39.8919) ccw
  line L1399 (6.3912, 39.8678) -> (6.5993, 40.3702)
  arc A1401 (6.5993, 40.3702) -> (6.4829, 40.4184) centre (6.5411, 40.3943) ccw
  line L1400 (6.27, 39.8919) -> (6.27, 39.6828)
  arc A1402 (6.27, 39.6828) -> (6.396, 39.6828) centre (6.333, 39.6828) ccw
  line L1401 (6.396, 39.6828) -> (6.396, 39.8919)
  arc A1403 (6.396, 39.8919) -> (6.27, 39.8919) centre (6.333, 39.8919) ccw
  line L1402 (6.333, 39.6198) -> (7.6365, 39.6198)
  arc A1404 (7.6365, 39.6198) -> (7.6365, 39.7458) centre (7.6365, 39.6828) ccw
  line L1403 (7.6365, 39.7458) -> (6.333, 39.7458)
  arc A1405 (6.333, 39.7458) -> (6.333, 39.6198) centre (6.333, 39.6828) ccw
  line L1404 (7.5735, 39.6828) -> (7.5735, 39.557)
  arc A1406 (7.5735, 39.557) -> (7.6995, 39.557) centre (7.6365, 39.557) ccw
  line L1405 (7.6995, 39.557) -> (7.6995, 39.6828)
  arc A1407 (7.6995, 39.6828) -> (7.5735, 39.6828) centre (7.6365, 39.6828) ccw
  line L1406 (7.6365, 39.62) -> (6.333, 39.62)
  arc A1408 (6.333, 39.62) -> (6.333, 39.494) centre (6.333, 39.557) ccw
  line L1407 (6.333, 39.494) -> (7.6365, 39.494)
  arc A1409 (7.6365, 39.494) -> (7.6365, 39.62) centre (7.6365, 39.557) ccw
  line L1408 (6.27, 39.557) -> (6.27, 39.348)
  arc A1410 (6.27, 39.348) -> (6.396, 39.348) centre (6.333, 39.348) ccw
  line L1409 (6.396, 39.348) -> (6.396, 39.557)
  arc A1411 (6.396, 39.557) -> (6.27, 39.557) centre (6.333, 39.557) ccw
  line L1410 (6.2748, 39.3239) -> (6.4829, 38.8215)
  arc A1412 (6.4829, 38.8215) -> (6.5993, 38.8697) centre (6.5411, 38.8456) ccw
  line L1411 (6.5993, 38.8697) -> (6.3912, 39.3721)
  arc A1413 (6.3912, 39.3721) -> (6.2748, 39.3239) centre (6.333, 39.348) ccw
  line L1412 (6.4966, 38.8011) -> (6.8811, 38.4166)
  arc A1414 (6.8811, 38.4166) -> (6.9701, 38.5056) centre (6.9256, 38.4611) ccw
  line L1413 (6.9701, 38.5056) -> (6.5856, 38.8901)
  arc A1415 (6.5856, 38.8901) -> (6.4966, 38.8011) centre (6.5411, 38.8456) ccw
  line L1414 (6.9015, 38.4029) -> (7.4039, 38.1948)
  arc A1416 (7.4039, 38.1948) -> (7.4521, 38.3112) centre (7.428, 38.253) ccw
  line L1415 (7.4521, 38.3112) -> (6.9497, 38.5193)
  arc A1417 (6.9497, 38.5193) -> (6.9015, 38.4029) centre (6.9256, 38.4611) ccw
  line L1416 (9.0283, 34.2882) -> (9.0283, 34.7917)
  arc A1418 (9.0283, 34.7917) -> (8.9023, 34.7917) centre (8.9653, 34.7917) ccw
  line L1417 (8.9023, 34.7917) -> (8.9023, 34.2882)
  arc A1419 (8.9023, 34.2882) -> (9.0283, 34.2882) centre (8.9653, 34.2882) ccw
  line L1418 (9.0235, 34.8158) -> (8.8309, 35.2808)
  arc A1420 (8.8309, 35.2808) -> (8.7145, 35.2326) centre (8.7727, 35.2567) ccw
  line L1419 (8.7145, 35.2326) -> (8.9071, 34.7676)
  arc A1421 (8.9071, 34.7676) -> (9.0235, 34.8158) centre (8.9653, 34.7917) ccw
  line L1420 (8.8172, 35.3012) -> (8.4612, 35.6572)
  arc A1422 (8.4612, 35.6572) -> (8.3722, 35.5682) centre (8.4167, 35.6127) ccw
  line L1421 (8.3722, 35.5682) -> (8.7282, 35.2122)
  arc A1423 (8.7282, 35.2122) -> (8.8172, 35.3012) centre (8.7727, 35.2567) ccw
  line L1422 (8.4408, 35.6709) -> (7.9758, 35.8635)
  arc A1424 (7.9758, 35.8635) -> (7.9276, 35.7471) centre (7.9517, 35.8053) ccw
  line L1423 (7.9276, 35.7471) -> (8.3926, 35.5545)
  arc A1425 (8.3926, 35.5545) -> (8.4408, 35.6709) centre (8.4167, 35.6127) ccw
  line L1424 (7.9517, 35.8683) -> (7.4482, 35.8683)
  arc A1426 (7.4482, 35.8683) -> (7.4482, 35.7423) centre (7.4482, 35.8053) ccw
  line L1425 (7.4482, 35.7423) -> (7.9517, 35.7423)
  arc A1427 (7.9517, 35.7423) -> (7.9517, 35.8683) centre (7.9517, 35.8053) ccw
  line L1426 (7.4241, 35.8635) -> (6.9591, 35.6709)
  arc A1428 (6.9591, 35.6709) -> (7.0073, 35.5545) centre (6.9832, 35.6127) ccw
  line L1427 (7.0073, 35.5545) -> (7.4723, 35.7471)
  arc A1429 (7.4723, 35.7471) -> (7.4241, 35.8635) centre (7.4482, 35.8053) ccw
  line L1428 (6.9387, 35.6572) -> (6.5827, 35.3012)
  arc A1430 (6.5827, 35.3012) -> (6.6717, 35.2122) centre (6.6272, 35.2567) ccw
  line L1429 (6.6717, 35.2122) -> (7.0277, 35.5682)
  arc A1431 (7.0277, 35.5682) -> (6.9387, 35.6572) centre (6.9832, 35.6127) ccw
  line L1430 (6.569, 35.2808) -> (6.3764, 34.8158)
  arc A1432 (6.3764, 34.8158) -> (6.4928, 34.7676) centre (6.4346, 34.7917) ccw
  line L1431 (6.4928, 34.7676) -> (6.6854, 35.2326)
  arc A1433 (6.6854, 35.2326) -> (6.569, 35.2808) centre (6.6272, 35.2567) ccw
  line L1432 (6.3716, 34.7917) -> (6.3716, 34.2882)
  arc A1434 (6.3716, 34.2882) -> (6.4976, 34.2882) centre (6.4346, 34.2882) ccw
  line L1433 (6.4976, 34.2882) -> (6.4976, 34.7917)
  arc A1435 (6.4976, 34.7917) -> (6.3716, 34.7917) centre (6.4346, 34.7917) ccw
  line L1434 (6.3764, 34.2641) -> (6.569, 33.7991)
  arc A1436 (6.569, 33.7991) -> (6.6854, 33.8473) centre (6.6272, 33.8232) ccw
  line L1435 (6.6854, 33.8473) -> (6.4928, 34.3123)
  arc A1437 (6.4928, 34.3123) -> (6.3764, 34.2641) centre (6.4346, 34.2882) ccw
  line L1436 (6.5827, 33.7787) -> (6.9387, 33.4227)
  arc A1438 (6.9387, 33.4227) -> (7.0277, 33.5117) centre (6.9832, 33.4672) ccw
  line L1437 (7.0277, 33.5117) -> (6.6717, 33.8677)
  arc A1439 (6.6717, 33.8677) -> (6.5827, 33.7787) centre (6.6272, 33.8232) ccw
  line L1438 (6.9591, 33.409) -> (7.4241, 33.2164)
  arc A1440 (7.4241, 33.2164) -> (7.4723, 33.3328) centre (7.4482, 33.2746) ccw
  line L1439 (7.4723, 33.3328) -> (7.0073, 33.5254)
  arc A1441 (7.0073, 33.5254) -> (6.9591, 33.409) centre (6.9832, 33.4672) ccw
  line L1440 (7.4482, 33.2116) -> (7.9517, 33.2116)
  arc A1442 (7.9517, 33.2116) -> (7.9517, 33.3376) centre (7.9517, 33.2746) ccw
  line L1441 (7.9517, 33.3376) -> (7.4482, 33.3376)
  arc A1443 (7.4482, 33.3376) -> (7.4482, 33.2116) centre (7.4482, 33.2746) ccw
  line L1442 (7.9758, 33.2164) -> (8.4408, 33.409)
  arc A1444 (8.4408, 33.409) -> (8.3926, 33.5254) centre (8.4167, 33.4672) ccw
  line L1443 (8.3926, 33.5254) -> (7.9276, 33.3328)
  arc A1445 (7.9276, 33.3328) -> (7.9758, 33.2164) centre (7.9517, 33.2746) ccw
  line L1444 (8.4612, 33.4227) -> (8.8172, 33.7787)
  arc A1446 (8.8172, 33.7787) -> (8.7282, 33.8677) centre (8.7727, 33.8232) ccw
  line L1445 (8.7282, 33.8677) -> (8.3722, 33.5117)
  arc A1447 (8.3722, 33.5117) -> (8.4612, 33.4227) centre (8.4167, 33.4672) ccw
  line L1446 (8.8309, 33.7991) -> (9.0235, 34.2641)
  arc A1448 (9.0235, 34.2641) -> (8.9071, 34.3123) centre (8.9653, 34.2882) ccw
  line L1447 (8.9071, 34.3123) -> (8.7145, 33.8473)
  arc A1449 (8.7145, 33.8473) -> (8.8309, 33.7991) centre (8.7727, 33.8232) ccw
  line L1448 (7.428, 17.87) -> (7.637, 17.87)
  arc A1450 (7.637, 17.87) -> (7.637, 17.996) centre (7.637, 17.933) ccw
  line L1449 (7.637, 17.996) -> (7.428, 17.996)
  arc A1451 (7.428, 17.996) -> (7.428, 17.87) centre (7.428, 17.933) ccw
  line L1450 (7.7, 17.933) -> (7.7, 19.2365)
  arc A1452 (7.7, 19.2365) -> (7.574, 19.2365) centre (7.637, 19.2365) ccw
  line L1451 (7.574, 19.2365) -> (7.574, 17.933)
  arc A1453 (7.574, 17.933) -> (7.7, 17.933) centre (7.637, 17.933) ccw
  line L1452 (7.637, 19.1735) -> (7.7628, 19.1735)
  arc A1454 (7.7628, 19.1735) -> (7.7628, 19.2995) centre (7.7628, 19.2365) ccw
  line L1453 (7.7628, 19.2995) -> (7.637, 19.2995)
  arc A1455 (7.637, 19.2995) -> (7.637, 19.1735) centre (7.637, 19.2365) ccw
  line L1454 (7.6998, 19.2365) -> (7.6998, 17.933)
  arc A1456 (7.6998, 17.933) -> (7.8258, 17.933) centre (7.7628, 17.933) ccw
  line L1455 (7.8258, 17.933) -> (7.8258, 19.2365)
  arc A1457 (7.8258, 19.2365) -> (7.6998, 19.2365) centre (7.7628, 19.2365) ccw
  line L1456 (7.7628, 17.87) -> (7.9719, 17.87)
  arc A1458 (7.9719, 17.87) -> (7.9719, 17.996) centre (7.9719, 17.933) ccw
  line L1457 (7.9719, 17.996) -> (7.7628, 17.996)
  arc A1459 (7.7628, 17.996) -> (7.7628, 17.87) centre (7.7628, 17.933) ccw
  line L1458 (7.996, 17.8748) -> (8.4984, 18.0829)
  arc A1460 (8.4984, 18.0829) -> (8.4502, 18.1993) centre (8.4743, 18.1411) ccw
  line L1459 (8.4502, 18.1993) -> (7.9478, 17.9912)
  arc A1461 (7.9478, 17.9912) -> (7.996, 17.8748) centre (7.9719, 17.933) ccw
  line L1460 (8.5188, 18.0966) -> (8.9033, 18.4811)
  arc A1462 (8.9033, 18.4811) -> (8.8143, 18.5701) centre (8.8588, 18.5256) ccw
  line L1461 (8.8143, 18.5701) -> (8.4298, 18.1856)
  arc A1463 (8.4298, 18.1856) -> (8.5188, 18.0966) centre (8.4743, 18.1411) ccw
  line L1462 (8.917, 18.5015) -> (9.1251, 19.0039)
  arc A1464 (9.1251, 19.0039) -> (9.0087, 19.0521) centre (9.0669, 19.028) ccw
  line L1463 (9.0087, 19.0521) -> (8.8006, 18.5497)
  arc A1465 (8.8006, 18.5497) -> (8.917, 18.5015) centre (8.8588, 18.5256) ccw
  line L1464 (9.1299, 19.028) -> (9.1299, 19.237)
  arc A1466 (9.1299, 19.237) -> (9.0039, 19.237) centre (9.0669, 19.237) ccw
  line L1465 (9.0039, 19.237) -> (9.0039, 19.028)
  arc A1467 (9.0039, 19.028) -> (9.1299, 19.028) centre (9.0669, 19.028) ccw
  line L1466 (9.0669, 19.3) -> (7.7634, 19.3)
  arc A1468 (7.7634, 19.3) -> (7.7634, 19.174) centre (7.7634, 19.237) ccw
  line L1467 (7.7634, 19.174) -> (9.0669, 19.174)
  arc A1469 (9.0669, 19.174) -> (9.0669, 19.3) centre (9.0669, 19.237) ccw
  line L1468 (7.8264, 19.237) -> (7.8264, 19.3628)
  arc A1470 (7.8264, 19.3628) -> (7.7004, 19.3628) centre (7.7634, 19.3628) ccw
  line L1469 (7.7004, 19.3628) -> (7.7004, 19.237)
  arc A1471 (7.7004, 19.237) -> (7.8264, 19.237) centre (7.7634, 19.237) ccw
  line L1470 (7.7634, 19.2998) -> (9.0669, 19.2998)
  arc A1472 (9.0669, 19.2998) -> (9.0669, 19.4258) centre (9.0669, 19.3628) ccw
  line L1471 (9.0669, 19.4258) -> (7.7634, 19.4258)
  arc A1473 (7.7634, 19.4258) -> (7.7634, 19.2998) centre (7.7634, 19.3628) ccw
  line L1472 (9.1299, 19.3628) -> (9.1299, 19.5719)
  arc A1474 (9.1299, 19.5719) -> (9.0039, 19.5719) centre (9.0669, 19.5719) ccw
  line L1473 (9.0039, 19.5719) -> (9.0039, 19.3628)
  arc A1475 (9.0039, 19.3628) -> (9.1299, 19.3628) centre (9.0669, 19.3628) ccw
  line L1474 (9.1251, 19.596) -> (8.917, 20.0984)
  arc A1476 (8.917, 20.0984) -> (8.8006, 20.0502) centre (8.8588, 20.0743) ccw
  line L1475 (8.8006, 20.0502) -> (9.0087, 19.5478)
  arc A1477 (9.0087, 19.5478) -> (9.1251, 19.596) centre (9.0669, 19.5719) ccw
  line L1476 (8.9033, 20.1188) -> (8.5188, 20.5033)
  arc A1478 (8.5188, 20.5033) -> (8.4298, 20.4143) centre (8.4743, 20.4588) ccw
  line L1477 (8.4298, 20.4143) -> (8.8143, 20.0298)
  arc A1479 (8.8143, 20.0298) -> (8.9033, 20.1188) centre (8.8588, 20.0743) ccw
  line L1478 (8.4984, 20.517) -> (7.996, 20.7251)
  arc A1480 (7.996, 20.7251) -> (7.9478, 20.6087) centre (7.9719, 20.6669) ccw
  line L1479 (7.9478, 20.6087) -> (8.4502, 20.4006)
  arc A1481 (8.4502, 20.4006) -> (8.4984, 20.517) centre (8.4743, 20.4588) ccw
  line L1480 (7.9719, 20.7299) -> (7.7628, 20.7299)
  arc A1482 (7.7628, 20.7299) -> (7.7628, 20.6039) centre (7.7628, 20.6669) ccw
  line L1481 (7.7628, 20.6039) -> (7.9719, 20.6039)
  arc A1483 (7.9719, 20.6039) -> (7.9719, 20.7299) centre (7.9719, 20.6669) ccw
  line L1482 (7.6998, 20.6669) -> (7.6998, 19.3634)
  arc A1484 (7.6998, 19.3634) -> (7.8258, 19.3634) centre (7.7628, 19.3634) ccw
  line L1483 (7.8258, 19.3634) -> (7.8258, 20.6669)
  arc A1485 (7.8258, 20.6669) -> (7.6998, 20.6669) centre (7.7628, 20.6669) ccw
  line L1484 (7.7628, 19.4264) -> (7.637, 19.4264)
  arc A1486 (7.637, 19.4264) -> (7.637, 19.3004) centre (7.637, 19.3634) ccw
  line L1485 (7.637, 19.3004) -> (7.7628, 19.3004)
  arc A1487 (7.7628, 19.3004) -> (7.7628, 19.4264) centre (7.7628, 19.3634) ccw
  line L1486 (7.7, 19.3634) -> (7.7, 20.6669)
  arc A1488 (7.7, 20.6669) -> (7.574, 20.6669) centre (7.637, 20.6669) ccw
  line L1487 (7.574, 20.6669) -> (7.574, 19.3634)
  arc A1489 (7.574, 19.3634) -> (7.7, 19.3634) centre (7.637, 19.3634) ccw
  line L1488 (7.637, 20.7299) -> (7.428, 20.7299)
  arc A1490 (7.428, 20.7299) -> (7.428, 20.6039) centre (7.428, 20.6669) ccw
  line L1489 (7.428, 20.6039) -> (7.637, 20.6039)
  arc A1491 (7.637, 20.6039) -> (7.637, 20.7299) centre (7.637, 20.6669) ccw
  line L1490 (7.4039, 20.7251) -> (6.9015, 20.517)
  arc A1492 (6.9015, 20.517) -> (6.9497, 20.4006) centre (6.9256, 20.4588) ccw
  line L1491 (6.9497, 20.4006) -> (7.4521, 20.6087)
  arc A1493 (7.4521, 20.6087) -> (7.4039, 20.7251) centre (7.428, 20.6669) ccw
  line L1492 (6.8811, 20.5033) -> (6.4966, 20.1188)
  arc A1494 (6.4966, 20.1188) -> (6.5856, 20.0298) centre (6.5411, 20.0743) ccw
  line L1493 (6.5856, 20.0298) -> (6.9701, 20.4143)
  arc A1495 (6.9701, 20.4143) -> (6.8811, 20.5033) centre (6.9256, 20.4588) ccw
  line L1494 (6.4829, 20.0984) -> (6.2748, 19.596)
  arc A1496 (6.2748, 19.596) -> (6.3912, 19.5478) centre (6.333, 19.5719) ccw
  line L1495 (6.3912, 19.5478) -> (6.5993, 20.0502)
  arc A1497 (6.5993, 20.0502) -> (6.4829, 20.0984) centre (6.5411, 20.0743) ccw
  line L1496 (6.27, 19.5719) -> (6.27, 19.3628)
  arc A1498 (6.27, 19.3628) -> (6.396, 19.3628) centre (6.333, 19.3628) ccw
  line L1497 (6.396, 19.3628) -> (6.396, 19.5719)
  arc A1499 (6.396, 19.5719) -> (6.27, 19.5719) centre (6.333, 19.5719) ccw
  line L1498 (6.333, 19.2998) -> (7.6365, 19.2998)
  arc A1500 (7.6365, 19.2998) -> (7.6365, 19.4258) centre (7.6365, 19.3628) ccw
  line L1499 (7.6365, 19.4258) -> (6.333, 19.4258)
  arc A1501 (6.333, 19.4258) -> (6.333, 19.2998) centre (6.333, 19.3628) ccw
  line L1500 (7.5735, 19.3628) -> (7.5735, 19.237)
  arc A1502 (7.5735, 19.237) -> (7.6995, 19.237) centre (7.6365, 19.237) ccw
  line L1501 (7.6995, 19.237) -> (7.6995, 19.3628)
  arc A1503 (7.6995, 19.3628) -> (7.5735, 19.3628) centre (7.6365, 19.3628) ccw
  line L1502 (7.6365, 19.3) -> (6.333, 19.3)
  arc A1504 (6.333, 19.3) -> (6.333, 19.174) centre (6.333, 19.237) ccw
  line L1503 (6.333, 19.174) -> (7.6365, 19.174)
  arc A1505 (7.6365, 19.174) -> (7.6365, 19.3) centre (7.6365, 19.237) ccw
  line L1504 (6.27, 19.237) -> (6.27, 19.028)
  arc A1506 (6.27, 19.028) -> (6.396, 19.028) centre (6.333, 19.028) ccw
  line L1505 (6.396, 19.028) -> (6.396, 19.237)
  arc A1507 (6.396, 19.237) -> (6.27, 19.237) centre (6.333, 19.237) ccw
  line L1506 (6.2748, 19.0039) -> (6.4829, 18.5015)
  arc A1508 (6.4829, 18.5015) -> (6.5993, 18.5497) centre (6.5411, 18.5256) ccw
  line L1507 (6.5993, 18.5497) -> (6.3912, 19.0521)
  arc A1509 (6.3912, 19.0521) -> (6.2748, 19.0039) centre (6.333, 19.028) ccw
  line L1508 (6.4966, 18.4811) -> (6.8811, 18.0966)
  arc A1510 (6.8811, 18.0966) -> (6.9701, 18.1856) centre (6.9256, 18.1411) ccw
  line L1509 (6.9701, 18.1856) -> (6.5856, 18.5701)
  arc A1511 (6.5856, 18.5701) -> (6.4966, 18.4811) centre (6.5411, 18.5256) ccw
  line L1510 (6.9015, 18.0829) -> (7.4039, 17.8748)
  arc A1512 (7.4039, 17.8748) -> (7.4521, 17.9912) centre (7.428, 17.933) ccw
  line L1511 (7.4521, 17.9912) -> (6.9497, 18.1993)
  arc A1513 (6.9497, 18.1993) -> (6.9015, 18.0829) centre (6.9256, 18.1411) ccw
  line L1512 (9.0283, 13.9682) -> (9.0283, 14.4717)
  arc A1514 (9.0283, 14.4717) -> (8.9023, 14.4717) centre (8.9653, 14.4717) ccw
  line L1513 (8.9023, 14.4717) -> (8.9023, 13.9682)
  arc A1515 (8.9023, 13.9682) -> (9.0283, 13.9682) centre (8.9653, 13.9682) ccw
  line L1514 (9.0235, 14.4958) -> (8.8309, 14.9608)
  arc A1516 (8.8309, 14.9608) -> (8.7145, 14.9126) centre (8.7727, 14.9367) ccw
  line L1515 (8.7145, 14.9126) -> (8.9071, 14.4476)
  arc A1517 (8.9071, 14.4476) -> (9.0235, 14.4958) centre (8.9653, 14.4717) ccw
  line L1516 (8.8172, 14.9812) -> (8.4612, 15.3372)
  arc A1518 (8.4612, 15.3372) -> (8.3722, 15.2482) centre (8.4167, 15.2927) ccw
  line L1517 (8.3722, 15.2482) -> (8.7282, 14.8922)
  arc A1519 (8.7282, 14.8922) -> (8.8172, 14.9812) centre (8.7727, 14.9367) ccw
  line L1518 (8.4408, 15.3509) -> (7.9758, 15.5435)
  arc A1520 (7.9758, 15.5435) -> (7.9276, 15.4271) centre (7.9517, 15.4853) ccw
  line L1519 (7.9276, 15.4271) -> (8.3926, 15.2345)
  arc A1521 (8.3926, 15.2345) -> (8.4408, 15.3509) centre (8.4167, 15.2927) ccw
  line L1520 (7.9517, 15.5483) -> (7.4482, 15.5483)
  arc A1522 (7.4482, 15.5483) -> (7.4482, 15.4223) centre (7.4482, 15.4853) ccw
  line L1521 (7.4482, 15.4223) -> (7.9517, 15.4223)
  arc A1523 (7.9517, 15.4223) -> (7.9517, 15.5483) centre (7.9517, 15.4853) ccw
  line L1522 (7.4241, 15.5435) -> (6.9591, 15.3509)
  arc A1524 (6.9591, 15.3509) -> (7.0073, 15.2345) centre (6.9832, 15.2927) ccw
  line L1523 (7.0073, 15.2345) -> (7.4723, 15.4271)
  arc A1525 (7.4723, 15.4271) -> (7.4241, 15.5435) centre (7.4482, 15.4853) ccw
  line L1524 (6.9387, 15.3372) -> (6.5827, 14.9812)
  arc A1526 (6.5827, 14.9812) -> (6.6717, 14.8922) centre (6.6272, 14.9367) ccw
  line L1525 (6.6717, 14.8922) -> (7.0277, 15.2482)
  arc A1527 (7.0277, 15.2482) -> (6.9387, 15.3372) centre (6.9832, 15.2927) ccw
  line L1526 (6.569, 14.9608) -> (6.3764, 14.4958)
  arc A1528 (6.3764, 14.4958) -> (6.4928, 14.4476) centre (6.4346, 14.4717) ccw
  line L1527 (6.4928, 14.4476) -> (6.6854, 14.9126)
  arc A1529 (6.6854, 14.9126) -> (6.569, 14.9608) centre (6.6272, 14.9367) ccw
  line L1528 (6.3716, 14.4717) -> (6.3716, 13.9682)
  arc A1530 (6.3716, 13.9682) -> (6.4976, 13.9682) centre (6.4346, 13.9682) ccw
  line L1529 (6.4976, 13.9682) -> (6.4976, 14.4717)
  arc A1531 (6.4976, 14.4717) -> (6.3716, 14.4717) centre (6.4346, 14.4717) ccw
  line L1530 (6.3764, 13.9441) -> (6.569, 13.4791)
  arc A1532 (6.569, 13.4791) -> (6.6854, 13.5273) centre (6.6272, 13.5032) ccw
  line L1531 (6.6854, 13.5273) -> (6.4928, 13.9923)
  arc A1533 (6.4928, 13.9923) -> (6.3764, 13.9441) centre (6.4346, 13.9682) ccw
  line L1532 (6.5827, 13.4587) -> (6.9387, 13.1027)
  arc A1534 (6.9387, 13.1027) -> (7.0277, 13.1917) centre (6.9832, 13.1472) ccw
  line L1533 (7.0277, 13.1917) -> (6.6717, 13.5477)
  arc A1535 (6.6717, 13.5477) -> (6.5827, 13.4587) centre (6.6272, 13.5032) ccw
  line L1534 (6.9591, 13.089) -> (7.4241, 12.8964)
  arc A1536 (7.4241, 12.8964) -> (7.4723, 13.0128) centre (7.4482, 12.9546) ccw
  line L1535 (7.4723, 13.0128) -> (7.0073, 13.2054)
  arc A1537 (7.0073, 13.2054) -> (6.9591, 13.089) centre (6.9832, 13.1472) ccw
  line L1536 (7.4482, 12.8916) -> (7.9517, 12.8916)
  arc A1538 (7.9517, 12.8916) -> (7.9517, 13.0176) centre (7.9517, 12.9546) ccw
  line L1537 (7.9517, 13.0176) -> (7.4482, 13.0176)
  arc A1539 (7.4482, 13.0176) -> (7.4482, 12.8916) centre (7.4482, 12.9546) ccw
  line L1538 (7.9758, 12.8964) -> (8.4408, 13.089)
  arc A1540 (8.4408, 13.089) -> (8.3926, 13.2054) centre (8.4167, 13.1472) ccw
  line L1539 (8.3926, 13.2054) -> (7.9276, 13.0128)
  arc A1541 (7.9276, 13.0128) -> (7.9758, 12.8964) centre (7.9517, 12.9546) ccw
  line L1540 (8.4612, 13.1027) -> (8.8172, 13.4587)
  arc A1542 (8.8172, 13.4587) -> (8.7282, 13.5477) centre (8.7727, 13.5032) ccw
  line L1541 (8.7282, 13.5477) -> (8.3722, 13.1917)
  arc A1543 (8.3722, 13.1917) -> (8.4612, 13.1027) centre (8.4167, 13.1472) ccw
  line L1542 (8.8309, 13.4791) -> (9.0235, 13.9441)
  arc A1544 (9.0235, 13.9441) -> (8.9071, 13.9923) centre (8.9653, 13.9682) ccw
  line L1543 (8.9071, 13.9923) -> (8.7145, 13.5273)
  arc A1545 (8.7145, 13.5273) -> (8.8309, 13.4791) centre (8.7727, 13.5032) ccw
  line L1544 (2.1578, 56.67) -> (2.337, 56.67)
  arc A1546 (2.337, 56.67) -> (2.337, 56.796) centre (2.337, 56.733) ccw
  line L1545 (2.337, 56.796) -> (2.1578, 56.796)
  arc A1547 (2.1578, 56.796) -> (2.1578, 56.67) centre (2.1578, 56.733) ccw
  line L1546 (2.4, 56.733) -> (2.4, 57.8865)
  arc A1548 (2.4, 57.8865) -> (2.274, 57.8865) centre (2.337, 57.8865) ccw
  line L1547 (2.274, 57.8865) -> (2.274, 56.733)
  arc A1549 (2.274, 56.733) -> (2.4, 56.733) centre (2.337, 56.733) ccw
  line L1548 (2.337, 57.8235) -> (2.4628, 57.8235)
  arc A1550 (2.4628, 57.8235) -> (2.4628, 57.9495) centre (2.4628, 57.8865) ccw
  line L1549 (2.4628, 57.9495) -> (2.337, 57.9495)
  arc A1551 (2.337, 57.9495) -> (2.337, 57.8235) centre (2.337, 57.8865) ccw
  line L1550 (2.3998, 57.8865) -> (2.3998, 56.733)
  arc A1552 (2.3998, 56.733) -> (2.5258, 56.733) centre (2.4628, 56.733) ccw
  line L1551 (2.5258, 56.733) -> (2.5258, 57.8865)
  arc A1553 (2.5258, 57.8865) -> (2.3998, 57.8865) centre (2.4628, 57.8865) ccw
  line L1552 (2.4628, 56.67) -> (2.6421, 56.67)
  arc A1554 (2.6421, 56.67) -> (2.6421, 56.796) centre (2.6421, 56.733) ccw
  line L1553 (2.6421, 56.796) -> (2.4628, 56.796)
  arc A1555 (2.4628, 56.796) -> (2.4628, 56.67) centre (2.4628, 56.733) ccw
  line L1554 (2.6662, 56.6748) -> (3.1134, 56.8601)
  arc A1556 (3.1134, 56.8601) -> (3.0652, 56.9765) centre (3.0893, 56.9183) ccw
  line L1555 (3.0652, 56.9765) -> (2.618, 56.7912)
  arc A1557 (2.618, 56.7912) -> (2.6662, 56.6748) centre (2.6421, 56.733) ccw
  line L1556 (3.1338, 56.8738) -> (3.4761, 57.2161)
  arc A1558 (3.4761, 57.2161) -> (3.3871, 57.3051) centre (3.4316, 57.2606) ccw
  line L1557 (3.3871, 57.3051) -> (3.0448, 56.9628)
  arc A1559 (3.0448, 56.9628) -> (3.1338, 56.8738) centre (3.0893, 56.9183) ccw
  line L1558 (3.4898, 57.2365) -> (3.6751, 57.6837)
  arc A1560 (3.6751, 57.6837) -> (3.5587, 57.7319) centre (3.6169, 57.7078) ccw
  line L1559 (3.5587, 57.7319) -> (3.3734, 57.2847)
  arc A1561 (3.3734, 57.2847) -> (3.4898, 57.2365) centre (3.4316, 57.2606) ccw
  line L1560 (3.6799, 57.7078) -> (3.6799, 57.887)
  arc A1562 (3.6799, 57.887) -> (3.5539, 57.887) centre (3.6169, 57.887) ccw
  line L1561 (3.5539, 57.887) -> (3.5539, 57.7078)
  arc A1563 (3.5539, 57.7078) -> (3.6799, 57.7078) centre (3.6169, 57.7078) ccw
  line L1562 (3.6169, 57.95) -> (2.4634, 57.95)
  arc A1564 (2.4634, 57.95) -> (2.4634, 57.824) centre (2.4634, 57.887) ccw
  line L1563 (2.4634, 57.824) -> (3.6169, 57.824)
  arc A1565 (3.6169, 57.824) -> (3.6169, 57.95) centre (3.6169, 57.887) ccw
  line L1564 (2.5264, 57.887) -> (2.5264, 58.0128)
  arc A1566 (2.5264, 58.0128) -> (2.4004, 58.0128) centre (2.4634, 58.0128) ccw
  line L1565 (2.4004, 58.0128) -> (2.4004, 57.887)
  arc A1567 (2.4004, 57.887) -> (2.5264, 57.887) centre (2.4634, 57.887) ccw
  line L1566 (2.4634, 57.9498) -> (3.6169, 57.9498)
  arc A1568 (3.6169, 57.9498) -> (3.6169, 58.0758) centre (3.6169, 58.0128) ccw
  line L1567 (3.6169, 58.0758) -> (2.4634, 58.0758)
  arc A1569 (2.4634, 58.0758) -> (2.4634, 57.9498) centre (2.4634, 58.0128) ccw
  line L1568 (3.6799, 58.0128) -> (3.6799, 58.1921)
  arc A1570 (3.6799, 58.1921) -> (3.5539, 58.1921) centre (3.6169, 58.1921) ccw
  line L1569 (3.5539, 58.1921) -> (3.5539, 58.0128)
  arc A1571 (3.5539, 58.0128) -> (3.6799, 58.0128) centre (3.6169, 58.0128) ccw
  line L1570 (3.6751, 58.2162) -> (3.4898, 58.6634)
  arc A1572 (3.4898, 58.6634) -> (3.3734, 58.6152) centre (3.4316, 58.6393) ccw
  line L1571 (3.3734, 58.6152) -> (3.5587, 58.168)
  arc A1573 (3.5587, 58.168) -> (3.6751, 58.2162) centre (3.6169, 58.1921) ccw
  line L1572 (3.4761, 58.6838) -> (3.1338, 59.0261)
  arc A1574 (3.1338, 59.0261) -> (3.0448, 58.9371) centre (3.0893, 58.9816) ccw
  line L1573 (3.0448, 58.9371) -> (3.3871, 58.5948)
  arc A1575 (3.3871, 58.5948) -> (3.4761, 58.6838) centre (3.4316, 58.6393) ccw
  line L1574 (3.1134, 59.0398) -> (2.6662, 59.2251)
  arc A1576 (2.6662, 59.2251) -> (2.618, 59.1087) centre (2.6421, 59.1669) ccw
  line L1575 (2.618, 59.1087) -> (3.0652, 58.9234)
  arc A1577 (3.0652, 58.9234) -> (3.1134, 59.0398) centre (3.0893, 58.9816) ccw
  line L1576 (2.6421, 59.2299) -> (2.4628, 59.2299)
  arc A1578 (2.4628, 59.2299) -> (2.4628, 59.1039) centre (2.4628, 59.1669) ccw
  line L1577 (2.4628, 59.1039) -> (2.6421, 59.1039)
  arc A1579 (2.6421, 59.1039) -> (2.6421, 59.2299) centre (2.6421, 59.1669) ccw
  line L1578 (2.3998, 59.1669) -> (2.3998, 58.0134)
  arc A1580 (2.3998, 58.0134) -> (2.5258, 58.0134) centre (2.4628, 58.0134) ccw
  line L1579 (2.5258, 58.0134) -> (2.5258, 59.1669)
  arc A1581 (2.5258, 59.1669) -> (2.3998, 59.1669) centre (2.4628, 59.1669) ccw
  line L1580 (2.4628, 58.0764) -> (2.337, 58.0764)
  arc A1582 (2.337, 58.0764) -> (2.337, 57.9504) centre (2.337, 58.0134) ccw
  line L1581 (2.337, 57.9504) -> (2.4628, 57.9504)
  arc A1583 (2.4628, 57.9504) -> (2.4628, 58.0764) centre (2.4628, 58.0134) ccw